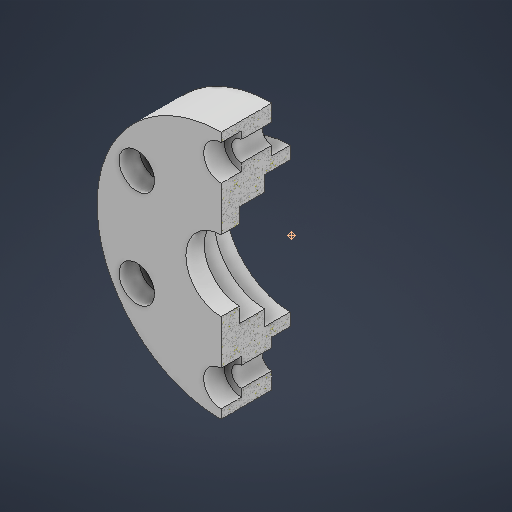
# Autodesk Inventor part: B2
Saved by Autodesk Inventor 2025.4 (Build 294407000, 407)
## iProperties
Created: 2026-05-15
Part Number: B2
Material: Generic
Document SubType Name: Modeling
Designer: VuQuan
Density: 1 g/cm^3
Appearance: Default
Author: VuQuan
Autodesk Inventor part; units mm, degrees
ref_plane "YZ Plane" through (0, 0, 0) normal (1, 0, 0) x (0, 1, 0)
ref_plane "XZ Plane" through (0, 0, 0) normal (0, 1, 0) x (-1, 0, 0)
ref_plane "XY Plane" through (0, 0, 0) normal (0, 0, 1) x (1, 0, 0)
sketch "Sketch1" plane through (0, 0, 0) normal (0, 0, 1) x (1, 0, 0)
  circle A0 centre (0, 0) radius 14
  circle A1 centre (0, 0) radius 20
  circle A2 centre (0, 0) radius 26
  circle A3 centre (0, 0) radius 31
  circle A4 centre (0, 0) radius 49
  circle A5 centre (0, 38.5) radius 7
  circle A6 centre (0, 38.5) radius 4
  dimension "d0" = 28
  dimension "d1" = 40
  dimension "d2" = 52
  dimension "d3" = 62
  dimension "d4" = 98
  dimension "d5" = 14
  dimension "d6" = 8
  dimension "d7" = 38.5
  constraints: 7 centre point, 6 coincident, 1 vertical alignment
  measures "d0" diameter of A0
  measures "d1" diameter of A1
  measures "d2" diameter of A2
  measures "d3" diameter of A3
  measures "d4" diameter of A4
  measures "d5" diameter of A5
  measures "d6" diameter of A6
  measures "d7" distance of point (0, 0) A5.centre
extrude "Extrusion1" add sketch "Sketch1" along normal blind 27.25 contours A0 | A1 | A2 | A3 | A4 | A5 | A6
extrude "Extrusion2" cut sketch "Sketch1" along normal through all contours A0
extrude "Extrusion3" cut sketch "Sketch1" along normal blind 7.25 contours A4 | A5 | A6
extrude "Extrusion4" cut sketch "Sketch1" along normal through all contours A6
extrude "Extrusion5" cut sketch "Sketch1" against normal blind 8 from surface at 27.25 contours A5
pattern_circular "Circular Pattern1" count 6 over 360 about axis through (0, 0, -10) along (0, 0, 1) of "Extrusion5", "Extrusion4"
extrude "Extrusion6" cut sketch "Sketch1" along normal blind 10 contours A0 | A1 | A2
extrude "Extrusion7" cut sketch "Sketch1" along normal blind 10 from surface at 10 contours A1
body "Solid1"
